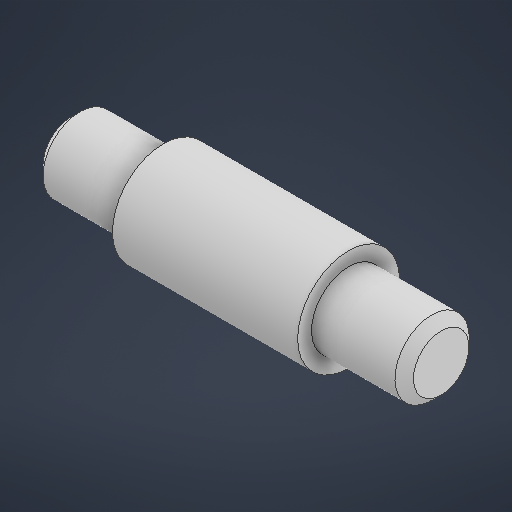
# Autodesk Inventor part: axle
Saved by Autodesk Inventor 2026 (Build 300175000, 175)
## iProperties
Created: 2025-05-07
Part Number: axle
Material: Generic
Document SubType Name: Modeling
Designer: Ritul Kumari
Density: 1 g/cm^3
Appearance: Default
Author: Ritul Kumari
Autodesk Inventor part; units mm, degrees
ref_plane "YZ Plane" through (0, 0, 0) normal (1, 0, 0) x (0, 1, 0)
ref_plane "XZ Plane" through (0, 0, 0) normal (0, 1, 0) x (-1, 0, 0)
ref_plane "XY Plane" through (0, 0, 0) normal (0, 0, 1) x (1, 0, 0)
sketch "Sketch1" plane through (0, 0, 0) normal (0, 0, 1) x (1, 0, 0)
  line L0 (-23.6137, 0) -> (-23.6137, 203.2)
  line L1 (-23.6137, 203.2) -> (484.3863, 203.2)
  line L2 (484.3863, 203.2) -> (484.3863, 279.4)
  line L3 (484.3863, 279.4) -> (1500.3863, 279.4)
  line L4 (1500.3863, 279.4) -> (1500.3863, 203.2)
  line L5 (1500.3863, 203.2) -> (2008.3863, 203.2)
  line L6 (2008.3863, 203.2) -> (2008.3863, 0)
  line L7 (2008.3863, 0) -> (-23.6137, 0)
  point P0 (0, 0)
  dimension "d0" = 203.2
  dimension "d1" = 508
  dimension "d2" = 76.2
  dimension "d3" = 1016
  dimension "d4" = 76.2
  dimension "d5" = 508
  constraints: 16 end point, 4 perpendicular, 2 point on line, 1 horizontal, 1 vertical
  measures "d0" distance of L0.start L0.end
  measures "d1" distance of L0.end L1.end
  measures "d2" distance of L1.end L2.end
  measures "d3" distance of L2.end L3.end
  measures "d4" distance of L3.end L4.end
  measures "d5" distance of L4.end L5.end
revolve "Revolution1" add sketch "Sketch1" angle 360 about axis through (2008.3863, 0, 0) along (-1, 0, 0)
chamfer "Chamfer1" distance 50.8 angle 45 2 edges at (-23.6137, -203.2, 0) (2008.3863, -203.2, 0)
body "Solid1"
